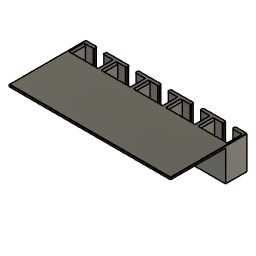
porte-cable v8 (Autodesk Fusion 360 design; units mm, degrees)
Autodesk Fusion 360 part; units mm, degrees
sketch "Esquisse1" plane through (0, 0, 0) normal (0, 0, 1) x (1, 0, 0)
  line L0 (51.25, -24.25) -> (-51.25, -24.25)
  line L1 (-51.25, -24.25) -> (-51.25, 24.25)
  line L2 (-51.25, 24.25) -> (51.25, 24.25)
  line L3 (51.25, 24.25) -> (51.25, -24.25)
  line L4 (51.25, -24.25) -> (-51.25, 24.25) construction
  line L5 (-51.25, -24.25) -> (51.25, 24.25) construction
  line L6 (-51.25, 10.75) -> (51.25, 10.75)
  line L7 (-49.25, 22.25) -> (-32.75, 22.25)
  line L8 (-32.75, 22.25) -> (-32.75, 13.75)
  line L9 (-32.75, 13.75) -> (-49.25, 13.75)
  line L10 (-49.25, 13.75) -> (-49.25, 22.25)
  line L11 (-28.75, 22.25) -> (-12.25, 22.25)
  line L12 (-12.25, 22.25) -> (-12.25, 13.75)
  line L13 (-12.25, 13.75) -> (-28.75, 13.75)
  line L14 (-28.75, 13.75) -> (-28.75, 22.25)
  line L15 (-8.25, 22.25) -> (8.25, 22.25)
  line L16 (8.25, 22.25) -> (8.25, 13.75)
  line L17 (8.25, 13.75) -> (-8.25, 13.75)
  line L18 (-8.25, 13.75) -> (-8.25, 22.25)
  line L19 (12.25, 22.25) -> (28.75, 22.25)
  line L20 (28.75, 22.25) -> (28.75, 13.75)
  line L21 (28.75, 13.75) -> (12.25, 13.75)
  line L22 (12.25, 13.75) -> (12.25, 22.25)
  line L23 (32.75, 22.25) -> (49.25, 22.25)
  line L24 (49.25, 22.25) -> (49.25, 13.75)
  line L25 (49.25, 13.75) -> (32.75, 13.75)
  line L26 (32.75, 13.75) -> (32.75, 22.25)
  line L27 (-43.875, 24.25) -> (-43.875, 22.25)
  line L28 (-38.125, 24.25) -> (-38.125, 22.25)
  line L29 (-41, 22.25) -> (-41, 13.75) construction
  line L30 (-20.5, 22.25) -> (-20.5, 13.75) construction
  line L31 (0, 22.25) -> (0, 13.75) construction
  line L32 (20.5, 22.25) -> (20.5, 13.75) construction
  line L33 (41, 22.25) -> (41, 13.75) construction
  line L34 (38.125, 24.25) -> (38.125, 22.25)
  line L35 (43.875, 24.25) -> (43.875, 22.25)
  line L36 (17.625, 24.25) -> (17.625, 22.25)
  line L37 (23.375, 24.25) -> (23.375, 22.25)
  line L38 (-2.875, 24.25) -> (-2.875, 22.25)
  line L39 (2.875, 24.25) -> (2.875, 22.25)
  line L40 (-23.375, 24.25) -> (-23.375, 22.25)
  line L41 (-17.625, 24.25) -> (-17.625, 22.25)
  line L42 (-43.875, 22.25) -> (-43.875, 13.75)
  line L43 (-38.125, 22.25) -> (-38.125, 13.75)
  line L44 (-23.375, 22.25) -> (-23.375, 13.75)
  line L45 (-17.625, 22.25) -> (-17.625, 13.75)
  line L46 (-2.875, 22.25) -> (-2.875, 13.75)
  line L47 (2.875, 22.25) -> (2.875, 13.75)
  line L48 (17.625, 22.25) -> (17.625, 13.75)
  line L49 (23.375, 22.25) -> (23.375, 13.75)
  line L50 (38.125, 22.25) -> (38.125, 13.75)
  line L51 (43.875, 22.25) -> (43.875, 13.75)
  dimension "d4" = 35
  dimension "d28" = 16.5
  dimension "d29" = 8.5
  dimension "d30" = 16.5
  dimension "d31" = 8.5
  dimension "d32" = 16.5
  dimension "d33" = 8.5
  dimension "d34" = 16.5
  dimension "d35" = 8.5
  dimension "d36" = 16.5
  dimension "d37" = 8.5
  dimension "d38" = 2
  dimension "d39" = 3
  dimension "d40" = 2
  dimension "d41" = 2
  dimension "d42" = 4
  dimension "d43" = 4
  dimension "d44" = 4
  dimension "d45" = 4
  dimension "d56" = 5.75
  dimension "d57" = 5.75
  dimension "d58" = 5.75
  dimension "d59" = 5.75
  dimension "d60" = 5.75
  constraint horizontal L0
  constraint perpendicular L0 L1
  constraint parallel L0 L2
  constraint parallel L1 L3
  constraint coincident L4 origin
  constraint coincident L5 origin
  constraint coincident L1 L6.start
  constraint coincident L3 L6.end
  constraint perpendicular L3 L6
  constraint horizontal L7
  constraint vertical L8
  constraint horizontal L9
  constraint vertical L10
  constraint horizontal L11
  constraint vertical L12
  constraint horizontal L13
  constraint vertical L14
  constraint horizontal L15
  constraint vertical L16
  constraint horizontal L17
  constraint vertical L18
  constraint horizontal L19
  constraint vertical L20
  constraint horizontal L21
  constraint vertical L22
  constraint horizontal L23
  constraint vertical L24
  constraint horizontal L25
  constraint vertical L26
  constraint collinear L7 L11
  constraint collinear L7 L15
  constraint collinear L7 L19
  constraint collinear L7 L23
  constraint coincident L2 L27.start
  constraint coincident L7 L27.end
  constraint perpendicular L7 L27
  constraint coincident L2 L28.start
  constraint coincident L7 L28.end
  constraint perpendicular L2 L28
  constraint midpoint L7 L29.start
  constraint midpoint L9 L29.end
  constraint midpoint L11 L30.start
  constraint midpoint L13 L30.end
  constraint midpoint L15 L31.start
  constraint midpoint L17 L31.end
  constraint midpoint L19 L32.start
  constraint midpoint L21 L32.end
  constraint midpoint L23 L33.start
  constraint midpoint L25 L33.end
  constraint coincident L2 L34.start
  constraint coincident L23 L34.end
  constraint perpendicular L23 L34
  constraint coincident L2 L35.start
  constraint coincident L23 L35.end
  constraint perpendicular L23 L35
  constraint coincident L2 L36.start
  constraint coincident L19 L36.end
  constraint perpendicular L19 L36
  constraint coincident L2 L37.start
  constraint coincident L19 L37.end
  constraint perpendicular L19 L37
  constraint coincident L2 L38.start
  constraint coincident L15 L38.end
  constraint perpendicular L15 L38
  constraint coincident L2 L39.start
  constraint coincident L15 L39.end
  constraint perpendicular L15 L39
  constraint coincident L2 L40.start
  constraint coincident L11 L40.end
  constraint perpendicular L11 L40
  constraint coincident L2 L41.start
  constraint coincident L11 L41.end
  constraint perpendicular L11 L41
  constraint symmetric L32 L36 L37
  constraint coincident L9 L42.end
  constraint perpendicular L9 L42
  constraint coincident L9 L43.end
  constraint perpendicular L9 L43
  constraint coincident L13 L44.end
  constraint perpendicular L13 L44
  constraint coincident L13 L45.end
  constraint perpendicular L13 L45
  constraint coincident L17 L46.end
  constraint perpendicular L17 L46
  constraint coincident L17 L47.end
  constraint perpendicular L17 L47
  constraint coincident L21 L48.end
  constraint perpendicular L21 L48
  constraint coincident L21 L49.end
  constraint perpendicular L21 L49
  constraint coincident L25 L50.end
  constraint perpendicular L25 L50
  constraint coincident L25 L51.end
  constraint perpendicular L25 L51
  measures "d4" distance of L0 L6
  measures "d28" distance of L7.start L7.end
  measures "d29" distance of L7.start L9.end
  measures "d30" distance of L11.start L11.end
  measures "d31" distance of L11.start L13.end
  measures "d32" distance of L15.start L15.end
  measures "d33" distance of L15.start L17.end
  measures "d34" distance of L19.start L19.end
  measures "d35" distance of L19.start L21.end
  measures "d36" distance of L23.start L23.end
  measures "d37" distance of L23.start L25.end
  measures "d38" distance of L2 L7
  measures "d39" distance of L6 L9
  measures "d40" distance of L1 L10
  measures "d41" distance of L3 L24
  measures "d42" distance of L8 L14
  measures "d43" distance of L12 L18
  measures "d44" distance of L16 L22
  measures "d45" distance of L20 L26
  measures "d56" distance of L27 L28
  measures "d57" distance of L40 L41
  measures "d58" distance of L38 L39
  measures "d59" distance of L36 L37
  measures "d60" distance of L34 L35
extrude "Extrusion1" add sketch "Esquisse1" against normal blind 3 contours L0 L1 L3 L6 makes body 1
extrude "Extrusion2" add 1 faces at (17.0833, -12.5833, -3) along direction (0, 0, -1) blind 2 on bodies 1 bodies 1
extrude "Extrusion3" cut 1 faces at (17.0833, -12.5833, -5) along direction (0, 0, 1) blind 4 on bodies 1 bodies 1
extrude "Extrusion4" add sketch "Esquisse1" along normal blind 12 separate body contours L1 L2 L3 L6 L7 L8 L9 L10 L11 L12 L13 L14 L15 L16 L17 L18 L19 L20 L21 L22 L23 L24 L25 L26 L27 L28 L34 L35 L36 L37 L38 L39 L40 L41 | L2 L23 L34 L35 | L2 L7 L27 L28 | L2 L19 L36 L37 | L2 L11 L40 L41 | L2 L15 L38 L39 makes body 2
extrude "Extrusion5" add sketch "Esquisse1" against normal blind 20 contours L1 L2 L3 L6 L7 L8 L9 L10 L11 L12 L13 L14 L15 L16 L17 L18 L19 L20 L21 L22 L23 L24 L25 L26 L27 L28 L34 L35 L36 L37 L38 L39 L40 L41 | L2 L23 L34 L35 | L2 L7 L27 L28 | L2 L19 L36 L37 | L2 L11 L40 L41 | L2 L15 L38 L39 bodies 1 2
extrude "Extrusion6" cut sketch "Esquisse1" along normal blind 12 and the other way blind 20 contours L2 L23 L34 L35 bodies 1
extrude "Extrusion7" cut sketch "Esquisse1" along normal blind 12 and the other way blind 20 contours L2 L7 L27 L28 | L2 L19 L36 L37 | L2 L11 L40 L41 | L2 L15 L38 L39 bodies 1
extrude "Extrusion8" cut 1 faces at (30.0833, 19.4167, 12) along direction (0, 0, -1) blind 12 on bodies 1 bodies 1
extrude "Extrusion9" add sketch "Esquisse1" against normal blind 21 contours L23 L24 L25 L51 bodies 1
extrude "Extrusion10" cut sketch "Esquisse1" against normal blind 20 contours L23 L24 L25 L51 bodies 1
extrude "Extrusion11" add 1 faces at (30.0833, 19.4167, -20) along direction (0, 0, -1) blind 1 on bodies 1 bodies 1
extrude "Extrusion12" add sketch "Esquisse1" against normal blind 21 contours L23 L25 L26 L50 bodies 1
extrude "Extrusion13" cut sketch "Esquisse1" against normal blind 20 contours L23 L25 L26 L50 bodies 1
extrude "Extrusion14" add sketch "Esquisse1" against normal blind 21 contours L19 L20 L21 L49 bodies 1
extrude "Extrusion15" cut sketch "Esquisse1" against normal blind 20 contours L19 L20 L21 L49 bodies 1
extrude "Extrusion16" add sketch "Esquisse1" against normal blind 21 contours L19 L21 L22 L48 bodies 1
extrude "Extrusion17" cut sketch "Esquisse1" against normal blind 20 contours L19 L21 L22 L48 bodies 1
extrude "Extrusion18" add sketch "Esquisse1" against normal blind 21 contours L15 L16 L17 L47 bodies 1
extrude "Extrusion19" cut sketch "Esquisse1" against normal blind 20 contours L15 L16 L17 L47 bodies 1
extrude "Extrusion20" add sketch "Esquisse1" against normal blind 21 contours L15 L17 L18 L46 bodies 1
extrude "Extrusion21" cut sketch "Esquisse1" against normal blind 20 contours L15 L17 L18 L46 bodies 1
extrude "Extrusion22" add sketch "Esquisse1" against normal blind 21 contours L11 L12 L13 L45 bodies 1
extrude "Extrusion23" cut sketch "Esquisse1" against normal blind 20 contours L11 L12 L13 L45 bodies 1
extrude "Extrusion24" add sketch "Esquisse1" against normal blind 21 contours L11 L13 L14 L44 bodies 1
extrude "Extrusion25" cut sketch "Esquisse1" against normal blind 20 contours L11 L13 L14 L44 bodies 1
extrude "Extrusion26" add sketch "Esquisse1" against normal blind 21 contours L7 L8 L9 L43 bodies 1
extrude "Extrusion27" cut sketch "Esquisse1" against normal blind 20 contours L7 L8 L9 L43 bodies 1
extrude "Extrusion28" add sketch "Esquisse1" against normal blind 21 contours L7 L9 L10 L42 bodies 1
extrude "Extrusion29" cut sketch "Esquisse1" against normal blind 20 contours L7 L9 L10 L42 bodies 1
fillet "Congé1" radius 0.5 10 edges at (43.875, 24.25, -10.5) (38.125, 24.25, -10.5) (23.375, 24.25, -10.5) (17.625, 24.25, -10.5) (2.875, 24.25, -10.5) (-2.875, 24.25, -10.5) (-17.625, 24.25, -10.5) (-23.375, 24.25, -10.5) (-38.125, 24.25, -10.5) (-43.875, 24.25, -10.5) on bodies 1
fillet "Congé2" radius 0.5 10 edges at (43.875, 22.25, -10) (38.125, 22.25, -10) (17.625, 22.25, -10) (-2.875, 22.25, -10) (23.375, 22.25, -10) (2.875, 22.25, -10) (-17.625, 22.25, -10) (-38.125, 22.25, -10) (-23.375, 22.25, -10) (-43.875, 22.25, -10) on bodies 1
fillet "Congé3" radius 0.2 6 edges at (-51.25, 0, 0) (0, -24.25, 0) (0, -24.25, -1) (51.25, 0, 0) (51.25, -6.75, -1) (-51.25, -6.75, -1) on bodies 1
chamfer "Chanfrein1" distance 1 angle 45 10 edges at (32.75, 18, 0) (49.25, 18, 0) (12.25, 18, 0) (28.75, 18, 0) (-8.25, 18, 0) (8.25, 18, 0) (-49.25, 18, 0) (-32.75, 18, 0) (-28.75, 18, 0) (-12.25, 18, 0) on bodies 1
fillet "Congé4" radius 0.5 10 edges at (38.125, 18.25, -20) (17.625, 18.25, -20) (-2.875, 18.25, -20) (-23.375, 18.25, -20) (-43.875, 18.25, -20) (43.875, 18.25, -20) (23.375, 18.25, -20) (2.875, 18.25, -20) (-17.625, 18.25, -20) (-38.125, 18.25, -20) on bodies 1
chamfer "Chanfrein2" distance 1 angle 45 5 edges at (41, 13.75, 0) (20.5, 13.75, 0) (0, 13.75, 0) (-20.5, 13.75, 0) (-41, 13.75, 0) on bodies 1
sketch "Esquisse2" plane through (0, 0, -1) normal (0, 0, -1) x (1, 0, 0)
  line L0 (51.05, -10.75) -> (51.05, 24.05)
  line L1 (51.05, 24.05) -> (-51.05, 24.05)
  line L2 (-51.05, 24.05) -> (-51.05, -10.75)
  line L3 (-51.05, -10.75) -> (51.05, -10.75)
  line L4 (35, -0.75) -> (-35, -0.75)
  line L5 (-35, -0.75) -> (-35, 19.25)
  line L6 (-35, 19.25) -> (35, 19.25)
  line L7 (35, 19.25) -> (35, -0.75)
  line L8 (-51.25, -10.75) -> (51.25, -10.75)
  dimension "d123" = 20
  dimension "d124" = 70
  dimension "d125" = 16.05
  dimension "d126" = 10
  constraint horizontal L4
  constraint vertical L5
  constraint horizontal L6
  constraint vertical L7
  measures "d123" distance of L4.start L6.end
  measures "d124" distance of L4.start L4.end
  measures "d125" distance of L0 L7
  measures "d126" distance of L4 L8
extrude "Extrusion30" cut sketch "Esquisse2" against normal blind 0.25 contours L4 L5 L6 L7 bodies 1
delete_face "DeleteFace1" 1 faces at (51.0967, -12.4755, -0.9945) on bodies 1
delete_face "DeleteFace2" 1 faces at (17.0884, -24.2407, -0.8601) on bodies 1
delete_face "DeleteFace3" 1 faces at (-51.0709, -12.5833, -0.9989) on bodies 1
extrude "Extrusion31" add 1 faces at (45.8333, -4.25, -1) along direction (0, 0, -1) blind 0.5 on bodies 1 bodies 1
extrude "Extrusion32" add 1 faces at (11.6667, -5.9167, -0.75) along direction (0, 0, -1) blind 0.5 on bodies 1 bodies 1
fillet "Congé5" radius 0.25 3 edges at (-51.25, -6.75, -1.5) (0, -24.25, -1.5) (51.25, -6.75, -1.5) on bodies 1
equation "d30 = d28"
equation "d31 = d29"
equation "d32 = d28"
equation "d33 = d29"
equation "d34 = d28"
equation "d35 = d29"
equation "d36 = d28"
equation "d37 = d29"
equation "d41 = d40"
equation "d43 = d42"
equation "d44 = d42"
equation "d45 = d42"
equation "d57 = d56"
equation "d58 = d56"
equation "d59 = d56"
equation "d60 = d56"
